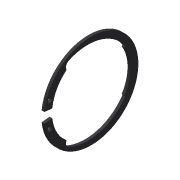
# Autodesk Inventor part: 3136 7009 59
Saved by Autodesk Inventor 2022 Beta2 (Build 260130000, 130) ContinuousBuild 0
## iProperties
Shininess: 0.0
Length Units: 11269
Angle Units: 11279
Time Units: 11290
Mass Units: 11283
Length Display Precision: 3
Angle Display Precision: 2
Compacted: True
Part Number: 3136 7009 59
Document SubType Name: Modeling
Description: Lock ring
Designer: Joe M
Engineer: Joe M
Density: 1 g/cm^3
Material: Generic
Appearance: Generic
Created: 2016-01-21
Density: 0.0
Volume: 0.0
Area: 0.0
PropertySet Name: Model Information
Control State: 0
Master: False
Checked Out: False
Last Check In Date: 2001-06-21
Last Check In By: iujhd
Title: Låsring
Author: Joe M
Autodesk Inventor part; units mm, degrees
ref_plane "YZ Plane" through (0, 0, 0) normal (1, 0, 0) x (0, 1, 0)
ref_plane "XZ Plane" through (0, 0, 0) normal (0, 1, 0) x (-1, 0, 0)
ref_plane "XY Plane" through (0, 0, 0) normal (0, 0, 1) x (1, 0, 0)
sketch "Sketch1" plane through (0, 0, 0) normal (0, 0, 1) x (1, 0, 0)
  line L0 (0, 0) -> (-75.2784, 0)
  line L1 (0, 28.5) -> (-2, 28.5)
  line L2 (-2, 28.5) -> (-2, 34.3)
  line L3 (-2, 34.3) -> (0, 34.3)
  line L4 (0, 34.3) -> (0, 28.5)
  point P0 (0, 0)
  dimension "d0" = 2
  dimension "d1" = 57
  dimension "d2" = 68.6
  constraints: 10 end point, 2 perpendicular, 1 coincident, 1 horizontal, 1 parallel, 1 vertical, 1 vertical alignment
  measures "d0" distance of L2.end L3.end
  measures "d1" diameter of L1 L0
  measures "d2" diameter of L3 L0
revolve "Revolution1" add sketch "Sketch1" angle 360 about axis through (0, 0, 0) along (-1, 0, 0)
sketch "Sketch2" plane through (0, 0, 0) normal (1, 0, 0) x (0, 0, -1)
  circle A0 centre (0, 0) radius 28.5 projected
  line L0 (0, 0) -> (15, 24.2332) construction
  line L1 (0, 0) -> (-15, 24.2332) construction
  line L2 (0, 0) -> (3.1, -28.3309) construction
  line L3 (0, 0) -> (-3.1, -28.3309) construction
  circle A1 centre (0, 0) radius 34.3 projected
  line L4 (3.1, -28.3309) -> (3.7309, -34.0965)
  line L5 (-3.1, -28.3309) -> (-3.7309, -34.0965)
  line L6 (15, 24.2332) -> (15.8503, 24.7596)
  line L7 (-15, 24.2332) -> (-15.8503, 24.7596)
  line L8 (0, 0) -> (22, -18.1177) construction
  line L9 (0, 0) -> (-22, -18.1177) construction
  circle A2 centre (0, 0) radius 31.8 construction
  line L10 (-22, -18.1177) -> (-23.8497, -18.3201)
  line L11 (22, -18.1177) -> (23.8497, -18.3201)
  arc A3 (-27.1979, -16.4377) -> (-23.8497, -18.3201) centre (-24.2087, -15.0396) ccw
  arc A4 (23.8497, -18.3201) -> (27.1979, -16.4377) centre (24.2087, -15.0396) ccw
  arc A5 (-15.8503, 24.7596) -> (-27.1979, -16.4377) centre (2.6227, -2.4902) ccw
  arc A6 (27.1979, -16.4377) -> (15.8503, 24.7596) centre (-2.6227, -2.4902) ccw
  circle A7 centre (0, 0) radius 31.4 construction
  line L12 (3.4154, -31.2137) -> (18.4181, -29.5721) construction
  circle A8 centre (9, -30.0826) radius 1.55
  circle A9 centre (-9, -30.0826) radius 1.55
  dimension "d4" = 30
  dimension "d5" = 6.2
  dimension "d6" = 1
  dimension "d7" = 44
  dimension "d8" = 2.5
  dimension "d9" = 32.9211
  dimension "d10" = 3.1
  dimension "d11" = 18
  constraints: 26 end point, 12 point on circle, 8 centre point, 7 tangent, 5 horizontal alignment, 5 perpendicular, 2 coincident, 2 collinear, 2 equal radius, 1 equal length, 1 midpoint, 8 other
  measures "d4" distance of L1.end L0.end
  measures "d5" distance of L3.end L2.end
  measures "d6" distance of L0.end L6.end
  measures "d7" distance of L9.end L8.end
  measures "d8" radial gap between concentric circles of A2 A1
  measures "d9" radius of A6
  measures "d10" diameter of A9
  measures "d11" distance of A9.centre A8.centre
extrude "Extrusion1" cut sketch "Sketch2" against normal through all contours A0 L6 A6 A4 L11 | A0 L10 A3 A5 L7 | L4 A1 L5 A0 | A8 | A9
body "Solid1"
